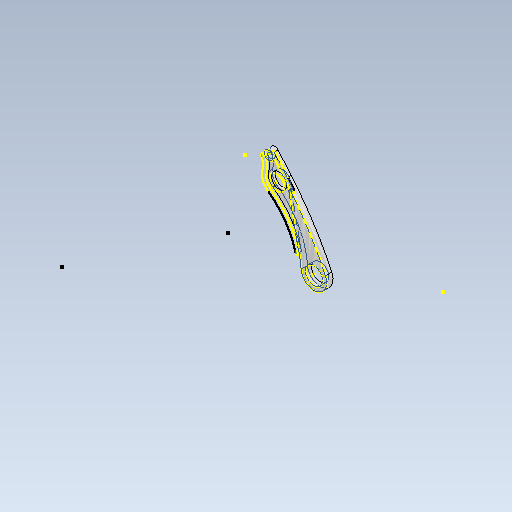
# Autodesk Inventor part: 揺動節
Saved by Autodesk Inventor 2020 (Build 240168000, 168)
## iProperties
Created: 2020-10-26
Part Number: 揺動節
Material: アルミニウム 7075
Document SubType Name: Modeling
Designer: AA19065
Density: 2.81 g/cm^3
Appearance: サテン - ブラシ仕上げ 重厚
Mass: 2.61501 g
Surface Area: 11.5679 cm^2
Volume: 0.930608 cm^3
Author: AA19065
Autodesk Inventor part; units mm, degrees
ref_plane "YZ Plane" through (0, 0, 0) normal (1, 0, 0) x (0, 1, 0)
ref_plane "XZ Plane" through (0, 0, 0) normal (0, 1, 0) x (-1, 0, 0)
ref_plane "XY Plane" through (0, 0, 0) normal (0, 0, 1) x (1, 0, 0)
sketch "スケッチ1" plane through (0, 0, 0) normal (0, 0, 1) x (1, 0, 0)
  line L0 (0, 0) -> (0, -25)
  line L1 (0, -25) -> (-17.5174, -20.86)
  line L2 (-17.5174, -20.86) -> (17.5174, -29.14)
  line L3 (17.5174, -29.14) -> (0, 0)
  circle A0 centre (0, 0) radius 5
  circle A1 centre (17.5174, -29.14) radius 4.025
  circle A2 centre (0, 0) radius 3.525
  circle A3 centre (17.5174, -29.14) radius 6
  line L4 (-4.899, 1) -> (-9.798, -23) construction
  circle A4 centre (-3.7755, 9.1288) radius 2
  line L5 (-2.2467, 10.4183) -> (3.8219, 3.2238)
  arc A5 (-4.8388, 1.2593) -> (-5.5656, 8.237) centre (-14.5164, 3.778) ccw
  circle A6 centre (0, -12) radius 4 construction
  arc A7 (11.5336, -29.5806) -> (-2.8846, -4.084) centre (-22.6724, -32.099) ccw
  arc A8 (22.9456, -26.5836) -> (3.8219, 3.2238) centre (-100.3634, -84.6572) ccw
  line L6 (5.375, 1.1681) -> (9.601, -19.535)
  line L7 (4.899, 1) -> (9.798, -23)
  arc A9 (5.375, 1.1681) -> (5.1695, 1.601) centre (4.3952, 0.9681) ccw
  arc A10 (9.601, -19.535) -> (10.4951, -23.3634) centre (78.1867, -5.535) ccw
  point P0 (3.8219, 3.2238)
  dimension "d0" = 36
  dimension "d1" = 18
  dimension "d2" = 34
  dimension "d3" = 10
  dimension "d4" = 8.05
  dimension "d5" = 7.05
  dimension "d6" = 12
  dimension "d7" = 4
  dimension "d8" = 10
  dimension "d9" = 34.2986
  dimension "d10" = 9.8788
  dimension "d11" = 43.7937
  dimension "d12" = 0.5
  dimension "d13" = 1
  dimension "d14" = 70
  constraints: 20 point on circle, 16 end point, 13 tangent, 11 centre point, 5 coincident, 1 collinear, 1 parallel, 3 other
  measures "d0" distance of L1.end L2.end
  measures "d1" distance of L0.end L1.end
  measures "d2" distance of L2.end L0.start
  measures "d3" diameter of A0
  measures "d4" diameter of A1
  measures "d5" diameter of A2
  measures "d6" diameter of A3
  measures "d7" diameter of A4
  measures "d8" radius of A5
  measures "d9" radius of A7
  measures "d10" distance of L0.start A4.centre
  measures "d11" distance of L2.end A4.centre
  measures "d12" distance between parallel lines of L6 L7
  measures "d13" radius of A9
  measures "d14" radius of A10
extrude "押し出し1" add sketch "スケッチ1" along normal blind 1.8 contours A2 L3 A0 L0 | L0 A0 L3 A2 | A0 L3 L7 A7 L0 | L0 A7 A0 | A0 L7 L3 | L7 A0 A8 A9 L6 L3 | L3 L6 A10 A7 L7 | A5 A4 L5 A0 | L6 A9 A8 A3 L3 | L3 A3 L2 A7 A10 L6 | L2 A3 A7 | A4 | A3 L2 A1 L3 | L3 A1 L2 A3
sketch "スケッチ3" plane through (0, 0, 1.8) normal (0, 0, 1) x (1, 0, 0)
  arc A0 (-4.8388, 1.2593) -> (-5.5656, 8.237) centre (-14.5164, 3.778) ccw projected
  arc A1 (-2.2467, 10.4183) -> (-5.5656, 8.237) centre (-3.7755, 9.1288) ccw projected
  line L0 (3.8219, 3.2238) -> (-2.2467, 10.4183) projected
  arc A2 (22.9456, -26.5836) -> (3.8219, 3.2238) centre (-100.3634, -84.6572) ccw projected
  arc A3 (11.5336, -29.5806) -> (22.9456, -26.5836) centre (17.5174, -29.14) ccw projected
  arc A4 (11.5336, -29.5806) -> (-2.8846, -4.084) centre (-22.6724, -32.099) ccw projected
  arc A5 (-4.8388, 1.2593) -> (-2.8846, -4.084) centre (0, 0) ccw projected
  circle A6 centre (0, 0) radius 3.525 projected
  circle A7 centre (17.5174, -29.14) radius 4.025 projected
  circle A8 centre (-3.7755, 9.1288) radius 2 projected
  arc A9 (5.375, 1.1681) -> (5.1695, 1.601) centre (4.3952, 0.9681) ccw projected
  line L1 (5.375, 1.1681) -> (9.601, -19.535) projected
  arc A10 (9.601, -19.535) -> (10.4951, -23.3634) centre (78.1867, -5.535) ccw projected
extrude "押し出し3" add sketch "スケッチ3" along normal blind 1.2 contours A1 A8 | A10 L1 A9 A2 A3 A4
fillet "フィレット2" radius 0.5 1 edges at (5.1695, 1.601, 2.4)
sketch "スケッチ4" plane through (0, 0, 0) normal (0, 0, -1) x (-1, 0, 0)
  arc A0 (5.5656, 8.237) -> (4.8388, 1.2593) centre (14.5164, 3.778) ccw projected
  arc A1 (5.5656, 8.237) -> (2.2467, 10.4183) centre (3.7755, 9.1288) ccw projected
  line L0 (-3.8219, 3.2238) -> (2.2467, 10.4183) projected
  arc A2 (-3.8219, 3.2238) -> (-22.9456, -26.5836) centre (100.3634, -84.6572) ccw projected
  arc A3 (-22.9456, -26.5836) -> (-11.5336, -29.5806) centre (-17.5174, -29.14) ccw projected
  arc A4 (2.8846, -4.084) -> (-11.5336, -29.5806) centre (22.6724, -32.099) ccw projected
  arc A5 (2.8846, -4.084) -> (4.8388, 1.2593) centre (0, 0) ccw projected
  circle A6 centre (0, 0) radius 3.525 projected
  circle A7 centre (-17.5174, -29.14) radius 4.025 projected
  line L1 (-9.601, -19.535) -> (-5.7393, -0.6167) projected
  arc A8 (-10.4951, -23.3634) -> (-9.601, -19.535) centre (-78.1867, -5.535) ccw projected
  arc A9 (-5.7393, -0.6167) -> (-6.6217, -0.2069) centre (-6.2292, -0.5167) ccw projected
  arc A10 (2.2467, 10.4183) -> (5.5656, 8.237) centre (3.7755, 9.1288) ccw projected
  line L2 (0.718, 11.7079) -> (-5.3507, 4.5133)
  arc A11 (-5.3507, 4.5133) -> (-24.7549, -25.7314) centre (100.3634, -84.6572) ccw
  arc A12 (4.0385, -5.7176) -> (-9.539, -29.7274) centre (22.6724, -32.099) ccw
  arc A13 (4.0385, -5.7176) -> (6.7743, 1.763) centre (0, 0) ccw
  arc A14 (7.3558, 7.3452) -> (6.7743, 1.763) centre (14.5164, 3.778) ccw
  arc A15 (7.3558, 7.3452) -> (5.5656, 8.237) centre (6.4607, 7.7911) ccw
  arc A16 (2.2467, 10.4183) -> (0.718, 11.7079) centre (1.4823, 11.0631) ccw
  arc A17 (-8.1915, 1.0323) -> (-6.6217, -0.2069) centre (-7.4066, 0.4127) ccw
  arc A18 (-5.7393, -0.6167) -> (-6.6217, -0.2069) centre (-6.2292, -0.5167) ccw projected
  arc A19 (-10.4951, -23.3634) -> (-8.5611, -23.8728) centre (-9.5281, -23.6181) ccw
  arc A20 (-10.4951, -23.3634) -> (-9.601, -19.535) centre (-78.1867, -5.535) ccw projected
  dimension "d27" = 2
  dimension "d28" = 2
  constraints: 18 point on circle, 8 centre point, 8 tangent, 2 end point, 3 other
  measures "d27" distance between parallel lines of L0 L2
  measures "d28" radial gap between concentric circles of A12 A4
sketch "スケッチ5" plane through (0, 0, 3) normal (0, 0, 1) x (1, 0, 0)
  arc A0 (-6.7743, 1.763) -> (-7.3558, 7.3452) centre (-14.5164, 3.778) ccw projected
  arc A1 (-5.5656, 8.237) -> (-7.3558, 7.3452) centre (-6.4607, 7.7911) ccw projected
  arc A2 (-6.7743, 1.763) -> (-4.0385, -5.7176) centre (0, 0) ccw projected
  arc A3 (8.5611, -23.8728) -> (-4.0385, -5.7176) centre (-22.6724, -32.099) ccw
  arc A4 (8.5611, -23.8728) -> (10.4951, -23.3634) centre (9.5281, -23.6181) ccw projected
  arc A5 (6.6217, -0.2069) -> (8.1915, 1.0323) centre (7.4066, 0.4127) ccw projected
  arc A6 (8.1915, 1.0323) -> (5.3507, 4.5133) centre (-100.3634, -84.6572) ccw
  line L0 (-0.718, 11.7079) -> (5.3507, 4.5133) projected
  arc A7 (-0.718, 11.7079) -> (-2.2467, 10.4183) centre (-1.4823, 11.0631) ccw projected
  circle A8 centre (-3.7755, 9.1288) radius 2 projected
  arc A9 (6.6217, -0.2069) -> (3.8219, 3.2238) centre (-100.3634, -84.6572) ccw projected
  line L1 (3.8219, 3.2238) -> (-2.2467, 10.4183) projected
  arc A10 (-5.5656, 8.237) -> (-2.2467, 10.4183) centre (-3.7755, 9.1288) ccw projected
  arc A11 (-4.8388, 1.2593) -> (-5.5656, 8.237) centre (-14.5164, 3.778) ccw projected
  arc A12 (-4.8388, 1.2593) -> (-2.8846, -4.084) centre (0, 0) ccw projected
  arc A13 (10.4951, -23.3634) -> (-2.8846, -4.084) centre (-22.6724, -32.099) ccw projected
  arc A14 (9.601, -19.535) -> (10.4951, -23.3634) centre (78.1867, -5.535) ccw projected
  line L2 (9.601, -19.535) -> (5.7393, -0.6167) projected
  arc A15 (6.6217, -0.2069) -> (5.7393, -0.6167) centre (6.2292, -0.5167) ccw projected
  circle A16 centre (0, 0) radius 3.525 projected
  circle A17 centre (17.5174, -29.14) radius 4.025 projected
  arc A18 (6.6217, -0.2069) -> (5.7393, -0.6167) centre (6.2292, -0.5167) ccw projected
  line L3 (5.7393, -0.6167) -> (9.601, -19.535) projected
  arc A19 (9.601, -19.535) -> (10.4951, -23.3634) centre (78.1867, -5.535) ccw projected
  arc A20 (11.5336, -29.5806) -> (10.4951, -23.3634) centre (-22.6724, -32.099) ccw projected
  arc A21 (11.5336, -29.5806) -> (22.9456, -26.5836) centre (17.5174, -29.14) ccw projected
  arc A22 (22.9456, -26.5836) -> (6.6217, -0.2069) centre (-100.3634, -84.6572) ccw projected
  constraints: 6 point on circle, 2 centre point, 2 other
equation "\"d0\" = d15"
equation "\"d1\" = d16"
equation "\"d2\" = d17"
equation "\"d15\" = 36"
equation "\"d16\" = 18"
equation "\"d17\" = 34"
